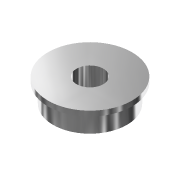
# Autodesk Inventor part: 30169-01
Saved by Autodesk Inventor 2014 (Build 180170000, 170)
## iProperties
Category: stocked
Created: 2013-07-17
Part Number: 30169-01
Material: Steel, Mild
Document SubType Name: Modeling
Designer: Edward
Density: 7.86 g/cm^3
Appearance: Chrome - Polished
Catalog Web Link: http://www.ebay.com/itm/100pcs-F608zz-Shielded-Model-Flange-Bearing-8-x-22-x-7mm-/251143541109?pt=BI_Heavy_Equipment_Parts&hash=item3a79525175
Description: 8x22x7mm flanged bearing
Stock Number: F608-ZZ
Project: Shapeoko
User Status: F
Vendor: Jinan Yuki Bearing Co., Ltd
Authority: NEED QUOTE FROM JINAN BEARING
Author: Edward
Subject: Motion
Comments: Inventables
Title: Flanged Bearing
Autodesk Inventor part; units mm, degrees
ref_plane "YZ Plane" through (0, 0, 0) normal (1, 0, 0) x (0, 1, 0)
ref_plane "XZ Plane" through (0, 0, 0) normal (0, 1, 0) x (-1, 0, 0)
ref_plane "XY Plane" through (0, 0, 0) normal (0, 0, 1) x (1, 0, 0)
sketch "Sketch1" plane through (0, 0, 0) normal (0, 0, 1) x (1, 0, 0)
  circle A0 centre (0, 0) radius 4
  circle A1 centre (0, 0) radius 11
  dimension "d0" = 8
  dimension "d1" = 22
  constraints: 2 centre point, 2 coincident
  measures "d0" diameter of A0
  measures "d1" diameter of A1
extrude "Extrusion1" add sketch "Sketch1" along normal blind 7
sketch "Sketch2" plane through (0, 0, 7) normal (0, 0, 1) x (1, 0, 0)
  circle A0 centre (0, 0) radius 11 projected
  circle A1 centre (0, 0) radius 12.5
  dimension "d4" = 25
  constraints: 1 centre point, 1 coincident
  measures "d4" diameter of A1
extrude "Extrusion2" add sketch "Sketch2" against normal blind 1.5
sketch "Sketch3" plane through (0, 0, 0) normal (0, 0, -1) x (-1, 0, 0)
  circle A0 centre (0, 0) radius 11 projected
  circle A1 centre (0, 0) radius 5.5937
  circle A2 centre (0, 0) radius 7.0513
  constraints: 2 centre point, 2 coincident
extrude "Extrusion3" cut sketch "Sketch3" against normal blind 0.1 contours A2
body "Solid1"
